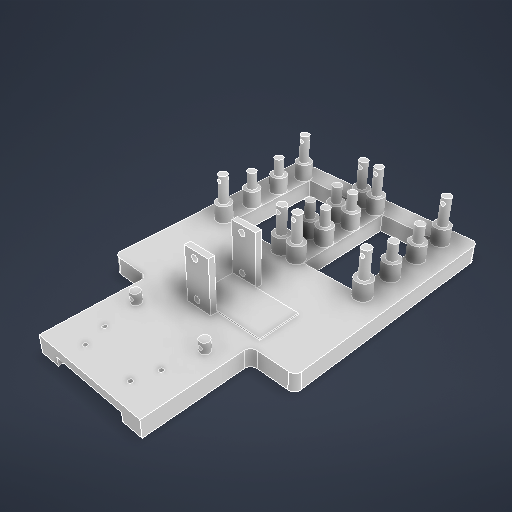
# Autodesk Inventor part: Lower_Chassis
Saved by Autodesk Inventor 2025 (Build 290162000, 162)
## iProperties
Created: 2024-06-03
Part Number: Lower_Chassis
Material: Generic
Document SubType Name: Modeling
Designer: Garfieldcmix
Density: 1 g/cm^3
Appearance: Default
Author: Garfieldcmix
Autodesk Inventor part; units mm, degrees
ref_plane "YZ Plane" through (0, 0, 0) normal (1, 0, 0) x (0, 1, 0)
ref_plane "XZ Plane" through (0, 0, 0) normal (0, 1, 0) x (-1, 0, 0)
ref_plane "XY Plane" through (0, 0, 0) normal (0, 0, 1) x (1, 0, 0)
derived "Car_Plan.ipt"
sketch "Car_Sketch" plane through (0, 0, 0) normal (0, 1, 0) x (-1, 0, 0)
  line L0 (0, 0) -> (94, 0)
  line L1 (0, 0) -> (0, 105)
  line L2 (94, 0) -> (94, 105)
  line L3 (0, 105) -> (20, 105)
  line L4 (20, 105) -> (20, 190)
  line L5 (20, 190) -> (74, 190)
  line L6 (74, 190) -> (74, 105)
  line L7 (74, 105) -> (94, 105)
  line L8 (-5, 68) -> (-5, 0)
  line L9 (-5, 0) -> (-32, 0)
  line L10 (-32, 0) -> (-32, 68)
  line L11 (-32, 68) -> (-5, 68)
  line L12 (47, 190) -> (47, 0) construction
  line L13 (126, 68) -> (99, 68)
  line L14 (99, 68) -> (99, 0)
  line L15 (126, 0) -> (126, 68)
  line L16 (99, 0) -> (126, 0)
  line L17 (-5, 34) -> (99, 34) construction
  line L18 (0, 95) -> (94, 95) construction
  line L19 (-5, 190) -> (-32, 190)
  line L20 (-32, 122) -> (-5, 122)
  line L21 (-32, 190) -> (-32, 122)
  line L22 (-5, 122) -> (-5, 190)
  line L23 (-5, 156) -> (99, 156) construction
  line L24 (126, 122) -> (99, 122)
  line L25 (126, 190) -> (126, 122)
  line L26 (99, 190) -> (126, 190)
  line L27 (99, 122) -> (99, 190)
  line L28 (0, 156) -> (47, 34) construction
  line L29 (94, 156) -> (47, 34) construction
  line L30 (0, 156) -> (-174.2341, 34) construction
  line L31 (-5, 34) -> (-174.2341, 34) construction
  line L32 (8.9873, 132.6713) -> (47, 141.55) construction
  line L33 (85.0127, 132.6713) -> (47, 141.55) construction
derived "Front_Bridge.ipt"
sketch "Front_Bridge_Base" plane through (0, 0, 0) normal (0, 1, 0) x (-1, 0, 0)
  circle A0 centre (0, 156) radius 1
  circle A1 centre (94, 156) radius 1
  line L0 (-5, 161) -> (-5, 151)
  line L1 (-5, 151) -> (29.5, 151)
  line L2 (99, 151) -> (99, 161)
  line L3 (99, 161) -> (90, 161)
  line L4 (4, 161) -> (22, 190)
  line L5 (22, 190) -> (72, 190)
  line L6 (72, 190) -> (90, 161)
  line L7 (0, 156) -> (94, 156) construction
  line L8 (4, 161) -> (-5, 161)
  line L9 (40.95, 172.3) -> (53.05, 172.3)
  line L10 (53.05, 172.3) -> (53.05, 149.9)
  line L11 (53.05, 149.9) -> (40.95, 149.9)
  line L12 (40.95, 149.9) -> (40.95, 172.3)
  line L13 (47, 156) -> (47, 149.9) construction
  line L14 (32, 151) -> (37, 144)
  line L15 (37, 144) -> (57, 144)
  line L16 (57, 144) -> (62, 151)
  line L17 (47, 156) -> (47, 144) construction
  line L18 (32, 151) -> (62, 151)
  line L19 (62, 151) -> (64.5, 151)
  line L20 (29.5, 151) -> (24.5, 126)
  line L21 (24.5, 126) -> (69.5, 126)
  line L22 (69.5, 126) -> (64.5, 151)
  line L23 (64.5, 151) -> (99, 151)
  line L24 (29.5, 151) -> (32, 151)
  line L25 (4, 161) -> (4, 151)
  line L26 (90, 161) -> (90, 151)
  circle A2 centre (32, 133) radius 1
  circle A3 centre (35, 143) radius 1
  line L27 (47, 156) -> (47, 126) construction
  circle A4 centre (59, 143) radius 1
  circle A5 centre (62, 133) radius 1
  line L28 (9, 169.0556) -> (9, 151)
  line L29 (84.8333, 151) -> (84.5992, 150.8961)
  line L30 (85, 169.0556) -> (85, 151)
  line L31 (26, 190) -> (26, 151)
  line L32 (68, 190) -> (68, 151)
  circle A6 centre (17, 157) radius 1.5
  circle A7 centre (17, 169) radius 1.5
  circle A8 centre (77, 157) radius 1.5
  circle A9 centre (77, 169) radius 1.5
sketch "Chassis_Base" plane through (0, 0, 0) normal (0, 1, 0) x (-1, 0, 0)
  line L0 (29.5, 151) -> (24.5, 126) projected
  line L1 (-5, 151) -> (29.5, 151) projected
  line L2 (20, 105) -> (20, 190) projected
  line L3 (24.5, 126) -> (69.5, 126) projected
  line L4 (69.5, 126) -> (64.5, 151) projected
  circle A0 centre (59, 143) radius 1 projected
  circle A1 centre (62, 133) radius 1 projected
  circle A2 centre (35, 143) radius 1 projected
  circle A3 centre (32, 133) radius 1 projected
  line L5 (74, 190) -> (74, 105) projected
  line L6 (74, 105) -> (94, 105) projected
  line L7 (0, 105) -> (20, 105) projected
  line L8 (0, 0) -> (0, 105) projected
  line L9 (0, 0) -> (94, 0) projected
  line L10 (94, 0) -> (94, 105) projected
  line L11 (64.5, 151) -> (99, 151) projected
  line L12 (62, 151) -> (64.5, 151) projected
  line L13 (32, 151) -> (62, 151) projected
  line L14 (29.5, 151) -> (32, 151) projected
  line L15 (19.9, 103.8) -> (19.9, 100.8) construction
  line L16 (19.9, 79) -> (40.75, 79) construction
  line L17 (52.75, 79) -> (52.75, 82)
  line L18 (52.75, 103.8) -> (40.75, 103.8)
  line L19 (52.75, 100.8) -> (19.9, 100.8)
  line L20 (52.75, 82) -> (19.9, 82)
  line L21 (19.9, 100.8) -> (19.9, 82)
  line L22 (19.9, 82) -> (19.9, 79) construction
  line L23 (52.75, 100.8) -> (52.75, 103.8)
  line L24 (52.75, 82) -> (52.75, 100.8)
  line L25 (40.75, 103.8) -> (40.75, 100.8)
  line L26 (40.75, 82) -> (40.75, 79)
  line L27 (40.75, 103.8) -> (19.9, 103.8) construction
  line L28 (40.75, 79) -> (52.75, 79)
  line L29 (47, 190) -> (47, 0) construction
  circle A4 centre (29, 117) radius 2.4
  circle A5 centre (65, 117) radius 2.4
  point P0 (20, 151)
  point P1 (74, 151)
  dimension "d31" = 1.2
  dimension "d32" = 24.8
  dimension "d33" = 19.9
  dimension "d34" = 32.85
  dimension "d35" = 18.8
  dimension "d36" = 3
  dimension "d41" = 12
  dimension "d50" = 4.8
  dimension "d51" = 12
  dimension "d52" = 18
  constraints: 28 end point, 27 perpendicular, 3 point on line, 3 vertical, 2 centre point, 1 collinear, 1 symmetric about line, 1 other
  measures "d31" distance from line of L7 L15.start
  measures "d32" distance of L16.start L15.start
  measures "d33" distance from line of L8 L16.start
  measures "d34" distance of L17.start L16.start
  measures "d35" distance of L20.end L15.end
  measures "d36" distance between parallel lines of L19 L18
  measures "d41" distance between parallel lines of L23 L25
  measures "d50" diameter of A4
  measures "d51" distance from line of A4.centre L7
  measures "d52" distance from line of L29 A4.centre
extrude "Chassis_Base_Extrusion" add sketch "Chassis_Base" along normal blind 8 contours L14 L13 L12 L4 L3 L0 | L0 L3 L4 L11 L5 L6 L10 L9 L8 L7 L2 L1 | L28 L26 L20 L17 | L20 L21 L19 L24 | L19 L25 L18 L23 | A4 | A5
extrude "Front_Bridge_Connector_Extrusion" cut sketch "Chassis_Base" along normal blind 4 contours L14 L13 L12 L4 L3 L0
sketch "Lego_Frame_Connector" plane through (0, 8, 0) normal (0, 1, 0) x (1, 0, 0)
  line L0 (5, -34) -> (-99, -34) construction
  circle A0 centre (-11.1, -42) radius 3.9
  circle A1 centre (-11.1, -26) radius 3.9
  circle A2 centre (-11.1, -58) radius 3.9
  circle A3 centre (-11.1, -10) radius 3.9
  circle A4 centre (-43.1, -58) radius 3.9
  circle A5 centre (-43.1, -42) radius 3.9
  circle A6 centre (-43.1, -26) radius 3.9
  circle A7 centre (-43.1, -10) radius 3.9
  line L1 (-11.1, -42) -> (-11.1, -26) construction
  line L2 (-11.1, -26) -> (-11.1, -10) construction
  line L3 (-11.1, -10) -> (-43.1, -10) construction
  line L4 (-43.1, -10) -> (-43.1, -26) construction
  line L5 (-43.1, -26) -> (-43.1, -42) construction
  line L6 (-43.1, -42) -> (-43.1, -58) construction
  line L7 (-43.1, -58) -> (-11.1, -58) construction
  line L8 (-11.1, -58) -> (-11.1, -42) construction
  line L9 (0, -105) -> (0, 0) projected
  circle A8 centre (-43.1, -58) radius 2.4
  circle A9 centre (-43.1, -42) radius 2.4
  circle A10 centre (-43.1, -26) radius 2.4
  circle A11 centre (-43.1, -10) radius 2.4
  circle A12 centre (-11.1, -10) radius 2.4
  circle A13 centre (-11.1, -26) radius 2.4
  circle A14 centre (-11.1, -42) radius 2.4
  circle A15 centre (-11.1, -58) radius 2.4
  line L10 (-39.2, -58) -> (-39.2, -10)
  line L11 (-15, -58) -> (-15, -10)
  line L12 (-15, -58) -> (-39.2, -58)
  line L13 (-39.2, -10) -> (-15, -10)
  line L14 (-47, -190) -> (-47, 0) construction
  circle A16 centre (-82.9, -42) radius 3.9
  circle A17 centre (-82.9, -26) radius 3.9
  circle A18 centre (-82.9, -58) radius 3.9
  circle A19 centre (-82.9, -10) radius 3.9
  circle A20 centre (-50.9, -58) radius 3.9
  circle A21 centre (-50.9, -42) radius 3.9
  circle A22 centre (-50.9, -26) radius 3.9
  circle A23 centre (-50.9, -10) radius 3.9
  line L15 (-82.9, -42) -> (-82.9, -26) construction
  line L16 (-82.9, -26) -> (-82.9, -10) construction
  line L17 (-82.9, -10) -> (-50.9, -10) construction
  line L18 (-50.9, -10) -> (-50.9, -26) construction
  line L19 (-50.9, -26) -> (-50.9, -42) construction
  line L20 (-50.9, -42) -> (-50.9, -58) construction
  line L21 (-50.9, -58) -> (-82.9, -58) construction
  line L22 (-82.9, -58) -> (-82.9, -42) construction
  circle A24 centre (-50.9, -58) radius 2.4
  circle A25 centre (-50.9, -42) radius 2.4
  circle A26 centre (-50.9, -26) radius 2.4
  circle A27 centre (-50.9, -10) radius 2.4
  circle A28 centre (-82.9, -10) radius 2.4
  circle A29 centre (-82.9, -26) radius 2.4
  circle A30 centre (-82.9, -42) radius 2.4
  circle A31 centre (-82.9, -58) radius 2.4
  line L23 (-54.8, -58) -> (-54.8, -10)
  line L24 (-79, -58) -> (-79, -10)
  line L25 (-79, -58) -> (-54.8, -58)
  line L26 (-54.8, -10) -> (-79, -10)
  point P0 (-11.1, -34)
  point P1 (-43.1, -34)
  point P2 (-94, 0)
  point P3 (-82.9, -34)
  point P4 (-50.9, -34)
  dimension "d8" = 7.8
  dimension "d9" = 7.8
  dimension "d10" = 7.8
  dimension "d13" = 7.8
  dimension "d6" = 7.8
  dimension "d7" = 7.8
  dimension "d11" = 7.8
  dimension "d12" = 7.8
  dimension "d14" = 16
  dimension "d15" = 32
  dimension "d19" = 4.8
  dimension "d20" = 4.8
  dimension "d21" = 4.8
  dimension "d22" = 4.8
  dimension "d23" = 4.8
  dimension "d24" = 4.8
  dimension "d25" = 4.8
  dimension "d26" = 4.8
  constraints: 48 end point, 24 centre point, 23 symmetric about line, 16 coincident, 8 collinear, 8 horizontal alignment, 8 point on line, 6 vertical, 4 perpendicular, 2 midpoint, 28 other
  measures "d6" diameter of A0
  measures "d7" diameter of A1
  measures "d11" diameter of A5
  measures "d12" diameter of A6
  measures "d14" distance of L1.start L7.end
  measures "d15" distance of L7.end L6.end
  measures "d19" diameter of A8
  measures "d20" diameter of A9
  measures "d21" diameter of A10
  measures "d22" diameter of A11
  measures "d23" diameter of A12
  measures "d24" diameter of A13
  measures "d25" diameter of A14
  measures "d26" diameter of A15
extrude "Hole_For_Differential_Extrusion" cut sketch "Lego_Frame_Connector" against normal through all contours L11 L12 L10 L13 | L25 L24 L26 L23
extrude "Lego_Frame_Connector_Extrusion" add sketch "Lego_Frame_Connector" along normal blind 8 contours A0 | A2 | A18 | A16 | A17 | A19 | A3 | A1 | A4 | A20 | A5 | A7 | A21 | A6 | A23 | A22 | A8 | A9 | A10 | A11 | A12 | A13 | A14 | A15 | A24 | A25 | A26 | A27 | A28 | A29 | A30 | A31
extrude "Lego_Frame_Connector_2_Extrusion" add sketch "Lego_Frame_Connector" along normal blind 15.8 contours A8 | A9 | A10 | A11 | A12 | A13 | A14 | A15 | A24 | A25 | A26 | A27 | A28 | A29 | A30 | A31
extrude "Motor_Base_Extrusion" add sketch "Chassis_Base" along normal blind 8.75 contours L20 L21 L19 L24
extrude "Motor_Holder_Extrusion" add sketch "Chassis_Base" along normal blind 32 contours L28 L26 L20 L17 | L19 L25 L18 L23
sketch "Motor_Screw_Hole" plane through (-40.75, 8, 79) normal (0, 0, -1) x (-1, 0, 0)
  circle A0 centre (6.95, 3.25) radius 1.5
  circle A1 centre (6.95, 20.75) radius 1.5
  line L0 (12, 0) -> (0, 0) projected
  line L1 (12, 0) -> (12, 24) projected
  point P0 (-40.75, -8)
  dimension "d42" = 3
  dimension "d43" = 3
  dimension "d44" = 3.25
  dimension "d45" = 5.05
  dimension "d46" = 17.5
  dimension "d47" = 5.05
  constraints: 2 centre point
  measures "d42" diameter of A0
  measures "d43" diameter of A1
  measures "d44" distance from line of L0 A0.centre
  measures "d45" distance from line of L1 A0.centre
  measures "d46" distance of A1.centre A0.centre
  measures "d47" distance from line of L1 A1.centre
extrude "Motor_Screw_Hole_Extrusion" cut sketch "Motor_Screw_Hole" against normal through all
sketch "1.5_Base_Screw" plane through (0, 8, 0) normal (0, 1, 0) x (1, 0, 0)
  circle A0 centre (-29, -117) radius 2.4 projected
  circle A1 centre (-65, -117) radius 2.4 projected
  point P0 (0, 0)
extrude "Pillar_Foundation_Extrusion" add sketch "1.5_Base_Screw" along normal blind 5
ref_plane "Foundation_Hole_Work_Plane" through (-29, 8, 119.4) normal (0, 0, 1) x (1, 0, 0)
sketch "Foundation_Hole_Sketch" plane through (-29, 8, 119.4) normal (0, 0, 1) x (1, 0, 0)
  line L0 (-33.6, 5) -> (-38.4, 5) construction
  line L1 (2.4, 5) -> (-2.4, 5) construction
  line L2 (-36, 5) -> (-36, 2.5) construction
  line L3 (0, 5) -> (0, 2.5) construction
  dimension "d208" = 2.5
  dimension "d209" = 2.5
  constraints: 4 end point, 2 midpoint, 2 perpendicular
  measures "d208" distance of L2.end L2.start
  measures "d209" distance of L3.end L3.start
hole "Foundation_Hole" at (-65, 10.5, 119.4) at (-29, 10.5, 119.4) direction (0, 0, -1) diameter 2 depth 4.8 tip angle 118
extrude "Pillar_Foundation_2_Extrusion" add sketch "Lego_Frame_Connector" along normal blind 20.8 contours A8 | A11 | A12 | A15 | A24 | A27 | A28 | A31
ref_plane "Foundation_2_Hole_Work_Plane" through (-43.1, 8, 60.4) normal (0, 0, -1) x (-1, 0, 0)
sketch "Foundation_2_Hole_Sketch" plane through (-43.1, 8, 60.4) normal (0, 0, -1) x (-1, 0, 0)
  line L0 (42.2, 20.8) -> (37.4, 20.8) construction
  line L1 (10.2, 20.8) -> (5.4, 20.8) construction
  line L2 (2.4, 20.8) -> (-2.4, 20.8) construction
  line L3 (-29.6, 20.8) -> (-34.4, 20.8) construction
  line L4 (39.8, 18.3) -> (39.8, 20.8) construction
  line L5 (7.8, 20.8) -> (7.8, 18.3) construction
  line L6 (0, 20.8) -> (0, 18.3) construction
  line L7 (-32, 20.8) -> (-32, 18.3) construction
  dimension "d204" = 2.5
  dimension "d205" = 2.5
  dimension "d206" = 2.5
  dimension "d207" = 2.5
  constraints: 8 end point, 4 midpoint, 4 perpendicular
  measures "d204" distance of L4.start L4.end
  measures "d205" distance of L5.end L5.start
  measures "d206" distance of L6.end L6.start
  measures "d207" distance of L7.end L7.start
hole "Foundation_2_Hole" at (-50.9, 26.3, 60.4) at (-43.1, 26.3, 60.4) at (-11.1, 26.3, 60.4) at (-82.9, 26.3, 60.4) direction (0, 0, -1) diameter 2 depth 4.8 tip angle 118
ref_plane "Foundation_3_Hole_Work_Plane" through (-11.1, 8, 12.4) normal (0, 0, -1) x (-1, 0, 0)
sketch "Foundation_3_Hole_Sketch" plane through (-11.1, 8, 12.4) normal (0, 0, -1) x (-1, 0, 0)
  line L0 (2.4, 20.8) -> (-2.4, 20.8) construction
  line L1 (34.4, 20.8) -> (29.6, 20.8) construction
  line L2 (42.2, 20.8) -> (37.4, 20.8) construction
  line L3 (74.2, 20.8) -> (69.4, 20.8) construction
  line L4 (71.8, 20.8) -> (71.8, 18.3) construction
  line L5 (39.8, 20.8) -> (39.8, 18.3) construction
  line L6 (32, 20.8) -> (32, 18.3) construction
  line L7 (0, 20.8) -> (0, 18.3) construction
  point P0 (-11.1, -8)
  dimension "d210" = 2.5
  dimension "d211" = 2.5
  dimension "d212" = 2.5
  dimension "d213" = 2.5
  constraints: 8 end point, 4 coincident, 4 midpoint, 4 perpendicular
  measures "d210" distance of L4.start L4.end
  measures "d211" distance of L5.start L5.end
  measures "d212" distance of L6.start L6.end
  measures "d213" distance of L7.start L7.end
hole "Foundation_3_Hole" at (-11.1, 26.3, 12.4) at (-43.1, 26.3, 12.4) at (-50.9, 26.3, 12.4) at (-82.9, 26.3, 12.4) direction (0, 0, -1) diameter 2 depth 4.8 tip angle 118
fillet "Fillet1" radius 3 6 edges at (-20, 4, 105) (0, 4, 105) (0, 4, 0) (-94, 4, 0) (-94, 4, 105) (-74, 4, 105)
offset faces "Size1" outward -0.15 faces at (-42.6924, 22.8351, 100.8) (-42.6924, 22.8351, 82)
offset faces "Size3" outward -0.2 faces at (-62.6311, 11.3333, 117.385) (-26.6311, 11.3333, 117.385) (-8.7311, 20.2667, 57.615) (-40.7311, 20.2667, 57.615) (-48.5311, 20.2667, 57.615) (-80.5311, 20.2667, 57.615) (-80.5311, 18.6, 41.615) (-48.5311, 18.6, 41.615) (-40.7311, 18.6, 41.615) (-8.7311, 18.6, 41.615) (-8.7078, 21.2, 26.1931) (-40.7078, 21.2, 26.1931) (-48.5078, 21.2, 26.1931) (-83.5677, 18.6, 23.6948) (-80.5311, 20.2667, 9.615) (-48.5311, 20.2667, 9.615) (-40.7311, 20.2667, 9.615) (-8.7311, 20.2667, 9.615)
body "Solid1"
